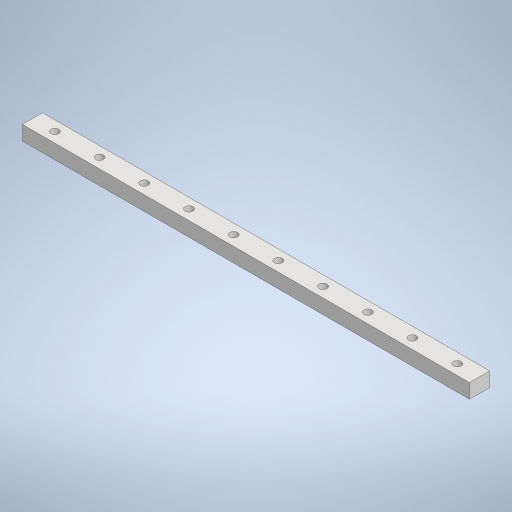
# Autodesk Inventor part: MGN9x200mm_rail
Saved by Autodesk Inventor 2024.1 (Build 281209000, 209)
## iProperties
Created: 2023-09-07
Part Number: MGN9x200mm_rail
Material: Generic
Document SubType Name: Modeling
Designer: l1534
Density: 1 g/cm^3
Appearance: Default
Author: l1534
Autodesk Inventor part; units mm, degrees
ref_plane "YZ Plane" through (0, 0, 0) normal (1, 0, 0) x (0, 1, 0)
ref_plane "XZ Plane" through (0, 0, 0) normal (0, 1, 0) x (-1, 0, 0)
ref_plane "XY Plane" through (0, 0, 0) normal (0, 0, 1) x (1, 0, 0)
sketch "Sketch1" plane through (0, 0, 0) normal (0, 1, 0) x (-1, 0, 0)
  line L0 (132.0119, -3.8652) -> (-67.9881, -3.8652)
  line L1 (-67.9881, -3.8652) -> (-67.9881, 5.1348)
  line L2 (-67.9881, 5.1348) -> (132.0119, 5.1348)
  line L3 (132.0119, 5.1348) -> (132.0119, -3.8652)
  point P0 (0, 0)
  dimension "d0" = 200
  dimension "d1" = 9
  constraints: 8 end point, 2 parallel, 1 horizontal, 1 perpendicular
  measures "d0" distance of L0.start L0.end
  measures "d1" distance of L0.end L1.end
extrude "Extrusion1" add sketch "Sketch1" along normal blind 6.5
sketch "Sketch2" plane through (0, 6.5, 0) normal (0, 1, 0) x (1, 0, 0)
  circle A0 centre (57.9881, -0.6348) radius 1.75
  line L0 (67.9881, 3.8652) -> (-132.0119, 3.8652) projected
  line L1 (67.9881, -5.1348) -> (67.9881, 3.8652) projected
  circle A1 centre (37.9881, -0.6348) radius 1.75
  circle A2 centre (17.9881, -0.6348) radius 1.75
  circle A3 centre (-2.0119, -0.6348) radius 1.75
  circle A4 centre (-22.0119, -0.6348) radius 1.75
  circle A5 centre (-42.0119, -0.6348) radius 1.75
  circle A6 centre (-62.0119, -0.6348) radius 1.75
  circle A7 centre (-82.0119, -0.6348) radius 1.75
  circle A8 centre (-102.0119, -0.6348) radius 1.75
  circle A9 centre (-122.0119, -0.6348) radius 1.75
  point P0 (0, 0)
  dimension "d4" = 3.5
  dimension "d5" = 4.5
  dimension "d6" = 10
  dimension "d9" = 20
  constraints: 10 centre point, 1 horizontal, 18 other
  measures "d4" diameter of A0
  measures "d5" distance from line of L0 A0.centre
  measures "d6" distance from line of L1 A0.centre
  measures "d9" distance of A0.centre A1.centre
extrude "Extrusion2" cut sketch "Sketch2" against normal through all
body "Solid1"
